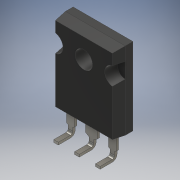
# Autodesk Inventor part: 56-0008-DOWN
Saved by Autodesk Inventor 2018 (Build 220112000, 112)
## iProperties
Created: 2018-05-30
Part Number: 56-0008-DOWN
Material: ABS Plastic
Document SubType Name: Modeling
Designer: Bradley
Density: 1.06 g/cm^3
Appearance: Smooth - Black
Author: Bradley
Autodesk Inventor part; units mm, degrees
ref_plane "YZ Plane" through (0, 0, 0) normal (1, 0, 0) x (0, 1, 0)
ref_plane "XY Plane" through (0, 0, 0) normal (0, 0, 1) x (1, 0, 0)
sketch "Sketch1" plane through (0, 0, 0) normal (0, 1, 0) x (-1, 0, 0)
  line L0 (7.8, -10.1) -> (-7.8, -10.1)
  line L1 (-7.8, -10.1) -> (-7.8, 10.1)
  line L2 (-7.8, 10.1) -> (7.8, 10.1)
  line L3 (7.8, 10.1) -> (7.8, -10.1)
  line L4 (7.8, -10.1) -> (-7.8, 10.1) construction
  line L5 (-7.8, -10.1) -> (7.8, 10.1) construction
  circle A0 centre (0, 4.59) radius 1.9
  arc A1 (-7.8, 2.59) -> (-7.8, 6.59) centre (-7.8, 4.59) ccw
  arc A2 (7.8, 6.59) -> (7.8, 2.59) centre (7.8, 4.59) ccw
  point P0 (0, 0)
  point P1 (0, 10.1)
  dimension "d0" = 20.2
  dimension "d1" = 15.6
  dimension "d39" = 3.8
  dimension "d40" = 5.51
  dimension "d41" = 4
  constraints: 12 end point, 6 point on line, 4 point on circle, 3 centre point, 3 midpoint, 2 horizontal alignment, 2 parallel, 1 equal radius, 1 horizontal, 1 perpendicular, 1 vertical alignment
  measures "d0" distance of L2.end L0.start
  measures "d1" distance of L1.end L2.end
  measures "d39" diameter of A0
  measures "d40" distance from line of A0.centre L2
  measures "d41" distance of A2.end A2.start
extrude "Extrusion6" add sketch "Sketch1" along normal blind 2
extrude "Extrusion7" add sketch "Sketch1" against normal blind 3 draft -7 contours L0 L1 A1 L2 L3 A2
ref_plane "Work Plane1" through (0, -0.4, 0) normal (0, 1, 0) x (-1, 0, 0)
sketch "Sketch4" plane through (0, -0.4, 0) normal (0, 1, 0) x (-1, 0, 0)
  line L0 (-7.8, -10.1) -> (7.8, -10.1) projected
  line L1 (-7.4316, -9.7316) -> (7.4316, -9.7316) projected
  line L2 (6.46, -9.7316) -> (6.46, -13.8691)
  line L3 (6.46, -13.8691) -> (6.06, -14.1)
  line L4 (6.06, -14.1) -> (6.06, -20.1)
  line L5 (4.86, -20.1) -> (4.86, -14.1)
  line L6 (4.86, -14.1) -> (4.46, -13.8691)
  line L7 (4.46, -13.8691) -> (4.46, -9.7316)
  line L8 (6.06, -20.1) -> (4.86, -20.1)
  line L9 (6.46, -9.7316) -> (4.46, -9.7316)
  line L10 (0, 0) -> (0, -9.7316) construction
  line L11 (-6.46, -9.7316) -> (-6.46, -13.8691)
  line L12 (-6.46, -13.8691) -> (-6.06, -14.1)
  line L13 (-6.06, -14.1) -> (-6.06, -20.1)
  line L14 (-4.86, -20.1) -> (-4.86, -14.1)
  line L15 (-4.86, -14.1) -> (-4.46, -13.8691)
  line L16 (-4.46, -13.8691) -> (-4.46, -9.7316)
  line L17 (-6.06, -20.1) -> (-4.86, -20.1)
  line L18 (-6.46, -9.7316) -> (-4.46, -9.7316)
  line L19 (1.5, -9.7316) -> (1.5, -13.5804)
  line L20 (1.5, -13.5804) -> (0.6, -14.1)
  line L21 (0.6, -14.1) -> (0.6, -20.1)
  line L22 (0.6, -20.1) -> (-0.6, -20.1)
  line L23 (-0.6, -20.1) -> (-0.6, -14.1)
  line L24 (-0.6, -14.1) -> (-1.5, -13.5804)
  line L25 (-1.5, -13.5804) -> (-1.5, -9.7316)
  line L26 (1.5, -9.7316) -> (-1.5, -9.7316)
  line L27 (6.46, -14.9775) -> (-6.46, -14.9775)
  circle A0 centre (0, 4.59) radius 1.9 projected
  point P0 (5.46, -20.1)
  point P1 (-5.46, -20.1)
  dimension "d46" = 2
  dimension "d47" = 1.2
  dimension "d48" = 4
  dimension "d51" = 120
  dimension "d53" = 6
  dimension "d54" = 5.46
  dimension "d55" = 3
  dimension "d66" = 19.5675
  constraints: 52 end point, 9 symmetric about line, 8 equal length, 6 perpendicular, 6 point on line, 5 parallel, 3 collinear, 3 midpoint, 1 horizontal, 1 vertical
  measures "d46" distance between parallel lines of L7 L2
  measures "d47" distance between parallel lines of L5 L4
  measures "d48" distance from line of L3.end L0
  measures "d51" angle of L6 L3
  measures "d53" distance of L3.end L4.end
  measures "d54" horizontal distance of L10.end point (5.46, -20.1)
  measures "d55" distance between parallel lines of L25 L19
  measures "d66" distance from line of L27 A0.centre
extrude "Extrusion4" add sketch "Sketch4" against normal blind 0.635 contours L11 L1 L16 L0 | L0 L16 L15 L14 L27 L13 L12 L11 | L25 L1 L19 L0 | L0 L19 L20 L21 L27 L23 L24 L25 | L27 L14 L17 L13 | L7 L1 L2 L0 | L0 L2 L3 L4 L27 L5 L6 L7 | L27 L21 L22 L23 | L27 L4 L8 L5
sketch "Sketch6" plane through (0, 2, 0) normal (0, 1, 0) x (1, 0, 0)
  circle A0 centre (0, -4.59) radius 1.9 projected
  line L0 (7.8, -10.1) -> (7.8, 10.1) projected
  line L1 (7.8, 10.1) -> (-7.8, 10.1) projected
  line L2 (-7.8, 10.1) -> (-7.8, -10.1) projected
  line L3 (-7.8, -10.1) -> (7.8, -10.1) projected
  line L4 (6.75, 4.8) -> (-6.75, 4.8)
  line L5 (-6.75, 4.8) -> (-6.75, -8.2)
  arc A1 (-6.75, -8.2) -> (-5.75, -9.2) centre (-5.75, -8.2) ccw
  line L6 (-5.75, -9.2) -> (-3.4, -9.2)
  line L7 (-3.4, -9.2) -> (-3, -9.6)
  line L8 (-3, -9.6) -> (3, -9.6)
  line L9 (3, -9.6) -> (3.4, -9.2)
  line L10 (3.4, -9.2) -> (5.75, -9.2)
  arc A2 (5.75, -9.2) -> (6.75, -8.2) centre (5.75, -8.2) ccw
  line L11 (6.75, -8.2) -> (6.75, 4.8)
  circle A3 centre (0, -4.59) radius 3
  point P0 (0, 0)
  point P1 (0, -9.6)
  point P2 (0, 4.8)
  dimension "d56" = 13.5
  dimension "d57" = 0.9
  dimension "d58" = 14
  dimension "d59" = 6
  dimension "d60" = 1
  dimension "d61" = 0.4
  dimension "d62" = 6
  constraints: 16 end point, 5 perpendicular, 4 point on circle, 4 tangent, 3 centre point, 2 midpoint, 2 point on line, 2 vertical alignment, 1 coincident, 1 equal radius, 1 horizontal, 1 parallel
  measures "d56" distance of L4.start L4.end
  measures "d57" distance between parallel lines of L6 L3
  measures "d58" distance between parallel lines of L4 L6
  measures "d59" diameter of A3
  measures "d60" radius of A1
  measures "d61" horizontal distance of L6.end L7.end
  measures "d62" distance of L7.end L8.end
extrude "Extrusion8" add sketch "Sketch6" along normal blind 0.01 contours L11 A2 L10 L9 L8 L7 L6 A1 L5 L4
bend part "Bend Part1" radius 1.25 angle 90 line through (-6.46, -0.4, -14.9775) along (1, 0, 0) centre toward (0, -1, 0) moving side (0, 0, -1) both sides no
body "Solid1"
body "Solid2"
